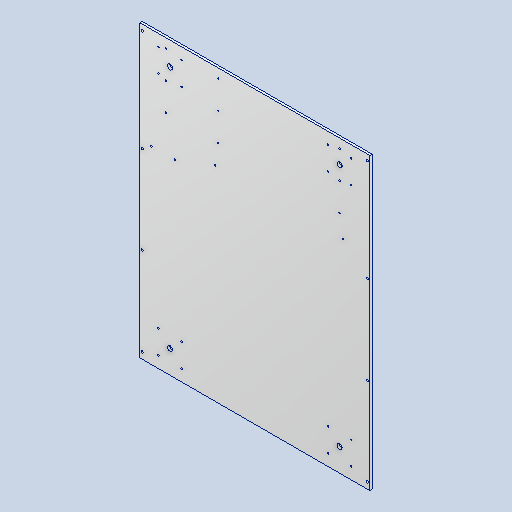
# Autodesk Inventor part: Base do fct bastidor
Saved by Autodesk Inventor 2026 (Build 300175050, 175E)
## iProperties
Created: 2025-08-25
Part Number: Base do fct bastidor
Material: Alumínio 6061
Document SubType Name: Modeling
Designer: Kedson Neves
Density: 2.7 g/cm^3
Appearance: Alumínio - Plano
Description: Base do fct bastidor
Author: Kedson Neves
Autodesk Inventor part; units mm, degrees
ref_plane "YZ Plane" through (0, 0, 0) normal (1, 0, 0) x (0, 1, 0)
ref_plane "XZ Plane" through (0, 0, 0) normal (0, 1, 0) x (-1, 0, 0)
ref_plane "XY Plane" through (0, 0, 0) normal (0, 0, 1) x (1, 0, 0)
sketch "Esboço1" plane through (0, 0, 0) normal (0, 0, 1) x (1, 0, 0)
  circle A0 centre (190.5217, 128.3199) radius 1.75
  circle A1 centre (-85.4783, 128.3199) radius 1.75
  circle A2 centre (-222.9771, 94.9699) radius 1.75
  circle A3 centre (-171.9771, 94.9699) radius 1.75
  circle A4 centre (-187.8891, -248.0369) radius 1.2295
  circle A5 centre (-187.8891, -233.0369) radius 1.2295
  circle A6 centre (-202.8891, -233.0369) radius 1.2295
  circle A7 centre (-202.8891, -248.0369) radius 1.2295
  circle A8 centre (188.1109, -248.0369) radius 1.2295
  circle A9 centre (203.1109, -248.0369) radius 1.2295
  circle A10 centre (188.1109, -233.0369) radius 1.2295
  circle A11 centre (203.1109, -233.0369) radius 1.2295
  circle A12 centre (203.1109, 298.1699) radius 1.2295
  circle A13 centre (188.1109, 298.1699) radius 1.2295
  circle A14 centre (188.1109, 283.1699) radius 1.2295
  circle A15 centre (203.1109, 283.1699) radius 1.2295
  circle A16 centre (-202.8891, 298.1699) radius 1.2295
  circle A17 centre (-187.8891, 298.1699) radius 1.2295
  circle A18 centre (-187.8891, 283.1699) radius 1.2295
  circle A19 centre (-202.8891, 283.1699) radius 1.2295
  line L0 (-169.1391, 123.1699) -> (-192.8891, 123.1699)
  line L1 (-192.8891, 123.1699) -> (-192.8891, 273.1699)
  line L2 (-192.8891, 273.1699) -> (-169.1391, 273.1699)
  line L3 (-169.1391, 273.1699) -> (-169.1391, 271.6699)
  line L4 (-169.1391, 271.6699) -> (-169.8891, 271.6699)
  line L5 (-169.8891, 271.6699) -> (-169.8891, 124.6699)
  line L6 (-169.8891, 124.6699) -> (-169.1391, 124.6699)
  line L7 (-169.1391, 124.6699) -> (-169.1391, 123.1699)
  line L8 (161.1979, 273.1699) -> (194.9479, 273.1699)
  line L9 (194.9479, 273.1699) -> (194.9479, 153.1699)
  line L10 (194.9479, 153.1699) -> (161.1979, 153.1699)
  line L11 (161.1979, 153.1699) -> (161.1979, 154.6699)
  line L12 (161.1979, 154.6699) -> (161.9479, 154.6699)
  line L13 (161.9479, 154.6699) -> (161.9479, 271.6699)
  line L14 (161.9479, 271.6699) -> (161.1979, 271.6699)
  line L15 (161.1979, 271.6699) -> (161.1979, 273.1699)
  arc A20 (248.1109, 311.1699) -> (246.1109, 313.1699) centre (246.1109, 311.1699) ccw
  line L16 (246.1109, 313.1699) -> (-245.8891, 313.1699)
  arc A21 (-245.8891, 313.1699) -> (-247.8891, 311.1699) centre (-245.8891, 311.1699) ccw
  line L17 (-247.8891, 311.1699) -> (-247.8891, -311.0369)
  arc A22 (-247.8891, -311.0369) -> (-245.8891, -313.0369) centre (-245.8891, -311.0369) ccw
  line L18 (-245.8891, -313.0369) -> (246.1109, -313.0369)
  arc A23 (246.1109, -313.0369) -> (248.1109, -311.0369) centre (246.1109, -311.0369) ccw
  line L19 (248.1109, -311.0369) -> (248.1109, 311.1699)
  circle A24 centre (-242.8891, 300.6699) radius 2.25
  circle A25 centre (243.1109, 300.6699) radius 2.25
  circle A26 centre (243.1109, 80.6699) radius 2.25
  circle A27 centre (243.1109, -299.3301) radius 2.25
  circle A28 centre (243.1109, -109.3301) radius 2.25
  circle A29 centre (-242.8891, -299.3301) radius 2.25
  circle A30 centre (-242.8891, -109.3301) radius 2.25
  circle A31 centre (-242.8891, 80.6699) radius 2.25
  line L20 (-58.9757, 153.1699) -> (-92.7257, 153.1699)
  line L21 (-92.7257, 153.1699) -> (-92.7257, 273.1699)
  line L22 (-92.7257, 273.1699) -> (-58.9757, 273.1699)
  line L23 (-58.9757, 273.1699) -> (-58.9757, 271.6699)
  line L24 (-58.9757, 271.6699) -> (-59.7257, 271.6699)
  line L25 (-59.7257, 271.6699) -> (-59.7257, 154.6699)
  line L26 (-59.7257, 154.6699) -> (-58.9757, 154.6699)
  line L27 (-58.9757, 154.6699) -> (-58.9757, 153.1699)
  line L28 (-231.6391, 273.1699) -> (-207.8891, 273.1699)
  line L29 (-207.8891, 273.1699) -> (-207.8891, 123.1699)
  line L30 (-207.8891, 123.1699) -> (-231.6391, 123.1699)
  line L31 (-231.6391, 123.1699) -> (-231.6391, 124.6699)
  line L32 (-231.6391, 124.6699) -> (-230.8891, 124.6699)
  line L33 (-230.8891, 124.6699) -> (-230.8891, 271.6699)
  line L34 (-230.8891, 271.6699) -> (-231.6391, 271.6699)
  line L35 (-231.6391, 271.6699) -> (-231.6391, 273.1699)
  point P0 (0, 0)
  point P1 (0.1552, -0.6774)
  constraints: 72 end point, 32 centre point, 8 point on circle
extrude "Extrusão1" add sketch "Esboço1" along normal blind 5 contours L0 L1 L2 L3 L4 L5 L6 L7 | L8 L9 L10 L11 L12 L13 L14 L15 | L19 A23 L18 A22 L17 A21 L16 A20 | L20 L21 L22 L23 L24 L25 L26 L27 | L28 L29 L30 L31 L32 L33 L34 L35
sketch "Esboço2" plane through (0, 0, 5) normal (0, 0, 1) x (1, 0, 0)
  line L0 (-211.7911, 303.4234) -> (-174.448, 303.4234)
  line L1 (-174.448, 303.4234) -> (-174.448, 277.9622)
  line L2 (-174.448, 277.9622) -> (-211.7911, 277.9622)
  line L3 (-211.7911, 277.9622) -> (-211.7911, 303.4234)
  line L4 (182.3897, 303.4234) -> (210.1357, 303.4234)
  line L5 (210.1357, 303.4234) -> (210.1357, 274.1618)
  line L6 (210.1357, 274.1618) -> (182.3897, 274.1618)
  line L7 (182.3897, 274.1618) -> (182.3897, 303.4234)
  line L8 (177.2667, -226.9528) -> (217.1375, -226.9528)
  line L9 (217.1375, -226.9528) -> (217.1375, -258.9103)
  line L10 (217.1375, -258.9103) -> (177.2667, -258.9103)
  line L11 (177.2667, -258.9103) -> (177.2667, -226.9528)
  line L12 (-216.7412, -223.4538) -> (-174.448, -223.4538)
  line L13 (-174.448, -223.4538) -> (-174.448, -261.7205)
  line L14 (-174.448, -261.7205) -> (-216.7412, -261.7205)
  line L15 (-216.7412, -261.7205) -> (-216.7412, -223.4538)
  point P0 (0, 0)
  constraints: 32 end point, 8 parallel, 4 horizontal, 4 perpendicular, 2 point on line
extrude "Extrusão2" add sketch "Esboço2" against normal blind 5
sketch "Esboço3" plane through (0, 0, 5) normal (0, 0, 1) x (1, 0, 0)
  line L0 (246.1109, 313.1699) -> (-245.8891, 313.1699) projected
  line L1 (-247.8891, 311.1699) -> (-247.8891, -311.0369) projected
  line L2 (0.1109, 313.1699) -> (0.1109, -313.0369)
  line L3 (-245.8891, -313.0369) -> (246.1109, -313.0369) projected
  line L4 (248.1109, -311.0369) -> (248.1109, 311.1699) projected
  line L5 (248.1109, 0.0665) -> (-247.8891, 0.0665)
  line L6 (248.1109, 311.1699) -> (248.1109, -311.0369)
  point P0 (0, 0)
  point P1 (-207.8891, 288.1699)
  point P2 (-157.8891, 288.1699)
  point P3 (-207.8891, 238.1699)
  point P4 (-157.8891, 238.1699)
  point P5 (208.1109, 288.1699)
  point P6 (158.1109, 288.1699)
  point P7 (208.1109, 238.1699)
  point P8 (158.1109, 238.1699)
  point P9 (-207.8891, -288.0369)
  point P10 (-157.8891, -288.0369)
  point P11 (-207.8891, -238.0369)
  point P12 (-157.8891, -238.0369)
  point P13 (158.1109, -238.0369)
  point P14 (208.1109, -238.0369)
  point P15 (158.1109, -288.0369)
  point P16 (208.1109, -288.0369)
  dimension "d4" = 50
  dimension "d5" = 25
  dimension "d6" = 40
  dimension "d7" = 50
  dimension "d8" = 50
  dimension "d9" = 0
  dimension "d10" = 50
  dimension "d11" = 40
  constraints: 12 symmetric about line, 6 end point, 4 midpoint
  measures "d4" distance of point (-157.889, 288.17) point (-207.889, 288.17)
  measures "d5" distance from line of L0 point (-207.889, 288.17)
  measures "d6" distance from line of L1 point (-207.889, 288.17)
  measures "d7" distance of point (-207.889, 238.17) point (-207.889, 288.17)
  measures "d8" distance of point (-157.889, 238.17) point (-207.889, 238.17)
  measures "d9" vertical distance of point (-207.889, 288.17) point (-157.889, 288.17)
  measures "d10" distance of point (-157.889, 238.17) point (-157.889, 288.17)
  measures "d11" distance from line of point (-207.889, 238.17) L1
hole "Furo1" at (-207.8891, 288.1699, 5) at (-157.8891, 288.1699, 5) at (-207.8891, 238.1699, 5) at (-157.8891, 238.1699, 5) at (158.1109, 238.1699, 5) at (208.1109, 238.1699, 5) at (158.1109, 288.1699, 5) at (208.1109, 288.1699, 5) at (-157.8891, -238.0369, 5) at (-207.8891, -238.0369, 5) at (-157.8891, -288.0369, 5) at (-207.8891, -288.0369, 5) at (208.1109, -288.0369, 5) at (158.1109, -288.0369, 5) at (208.1109, -238.0369, 5) at (158.1109, -238.0369, 5) direction (0, 0, -1) diameter 3.242 end through all thread size "M4x0.7" class "6H" standard "ISO Metric profile"
sketch "Esboço6" plane through (0, 0, 5) normal (0, 0, 1) x (1, 0, 0)
  circle A0 centre (183.1109, 263.1699) radius 4.188 projected
  circle A1 centre (-182.8891, 263.1699) radius 4.188 projected
  circle A2 centre (-182.8891, -263.0369) radius 4.188 projected
  circle A3 centre (183.1109, -263.0369) radius 4.188 projected
  point P0 (0, 0)
  constraints: 4 coincident
hole "Furo2" at (183.1109, -263.0369, 5) at (-182.8891, -263.0369, 5) at (183.1109, 263.1699, 5) at (-182.8891, 263.1699, 5) direction (0, 0, -1) diameter 11 end through all clearance for "Countersunk Flat Head Screw ISO 2009/7046" size "M10" standard "ISO"
sketch "Esboço7" plane through (0, 0, 0) normal (0, 0, -1) x (-1, 0, 0)
  circle A0 centre (191.8891, 233.1699) radius 4.7 construction
  circle A1 centre (191.8891, 293.1699) radius 4.7 construction
  circle A2 centre (191.8891, 173.1699) radius 4.7 construction
  line L0 (226.8891, 160.1699) -> (224.8891, 158.1699) construction
  line L1 (226.8891, 160.1699) -> (226.8891, 306.1699) construction
  line L2 (224.8891, 308.1699) -> (226.8891, 306.1699) construction
  line L3 (224.8891, 308.1699) -> (158.8891, 308.1699) construction
  line L4 (156.8891, 306.1699) -> (158.8891, 308.1699) construction
  line L5 (156.8891, 306.1699) -> (156.8891, 160.1699) construction
  line L6 (158.8891, 158.1699) -> (156.8891, 160.1699) construction
  line L7 (158.8891, 158.1699) -> (224.8891, 158.1699) construction
  circle A3 centre (78.7627, 233.1699) radius 4.7 construction
  circle A4 centre (78.7627, 293.1699) radius 4.7 construction
  circle A5 centre (78.7627, 173.1699) radius 4.7 construction
  line L8 (113.7627, 160.1699) -> (111.7627, 158.1699) construction
  line L9 (113.7627, 160.1699) -> (113.7627, 306.1699) construction
  line L10 (111.7627, 308.1699) -> (113.7627, 306.1699) construction
  line L11 (111.7627, 308.1699) -> (45.7627, 308.1699) construction
  line L12 (43.7627, 306.1699) -> (45.7627, 308.1699) construction
  line L13 (43.7627, 306.1699) -> (43.7627, 160.1699) construction
  line L14 (45.7627, 158.1699) -> (43.7627, 160.1699) construction
  line L15 (45.7627, 158.1699) -> (111.7627, 158.1699) construction
  circle A6 centre (-182.9109, 233.1699) radius 4.7 construction
  circle A7 centre (-182.9109, 293.1699) radius 4.7 construction
  circle A8 centre (-182.9109, 173.1699) radius 4.7 construction
  line L16 (-147.9109, 160.1699) -> (-149.9109, 158.1699) construction
  line L17 (-147.9109, 160.1699) -> (-147.9109, 306.1699) construction
  line L18 (-149.9109, 308.1699) -> (-147.9109, 306.1699) construction
  line L19 (-149.9109, 308.1699) -> (-215.9109, 308.1699) construction
  line L20 (-217.9109, 306.1699) -> (-215.9109, 308.1699) construction
  line L21 (-217.9109, 306.1699) -> (-217.9109, 160.1699) construction
  line L22 (-215.9109, 158.1699) -> (-217.9109, 160.1699) construction
  line L23 (-215.9109, 158.1699) -> (-149.9109, 158.1699) construction
  point P0 (0, 0)
  constraints: 9 coincident
hole "Furo3" at (182.9109, 293.1699, 0) at (182.9109, 233.1699, 0) at (182.9109, 173.1699, 0) at (-78.7627, 293.1699, 0) at (-78.7627, 233.1699, 0) at (-78.7627, 173.1699, 0) at (-191.8891, 293.1699, 0) at (-191.8891, 233.1699, 0) at (-191.8891, 173.1699, 0) direction (0, 0, 1) diameter 3.242 end through all thread size "M4x0.7" class "6H" standard "ISO Metric profile"
delete faces "Excluir1" heal yes whole lump no faces at (247.9726, 311.9006, 3.3333)
delete faces "Excluir2" heal yes whole lump no faces at (-247.5416, 312.2966, 3.3333)
delete faces "Excluir3" heal yes whole lump no faces at (248.022, -311.6264, 3.3333)
delete faces "Excluir4" heal yes whole lump no faces at (-247.7509, -311.7675, 3.3333)
